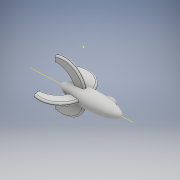
# Autodesk Inventor part: Rakete_Janneke
Saved by Autodesk Inventor 2017.3 (Build 213257000, 257)
## iProperties
Created: 2020-05-12
Part Number: Rakete_Janneke
Material: Generic
Document SubType Name: Modeling
Designer: Ole Simmering
Density: 1 g/cm^3
Appearance: Default
Author: Ole Simmering
Autodesk Inventor part; units mm, degrees
ref_plane "YZ Plane" through (0, 0, 0) normal (1, 0, 0) x (0, 1, 0)
ref_plane "XZ Plane" through (0, 0, 0) normal (0, 1, 0) x (-1, 0, 0)
ref_plane "XY Plane" through (0, 0, 0) normal (0, 0, 1) x (1, 0, 0)
sketch "Sketch1" plane through (0, 0, 0) normal (0, 0, 1) x (1, 0, 0)
  line L0 (23.379463, -14.591224) -> (429.779457, -14.591224) construction
  line L1 (429.779457, -14.591224) -> (429.779457, -319.391219) construction
  line L2 (429.779457, -319.391219) -> (23.379463, -319.391219) construction
  line L3 (23.379463, -319.391219) -> (23.379463, -14.591224) construction
  ellipse E0 centre (221, -186) end of major axis (94.610324, -191.310491) minor radius 34.213334 (347.389676, -180.689509) -> (94.610324, -191.310491) ccw
  line L4 (23.379463, -194.303384) -> (429.779457, -177.227754)
  ellipse E1 centre (221, -186) end of major axis (94.610324, -191.310491) minor radius 34.213334 (94.610324, -191.310491) -> (347.389676, -180.689509) ccw
  point P0 (0, 0)
  constraints: 4 point on line, 2 end point, 11 other
revolve "Revolution1" add sketch "Sketch1" angle 360 about axis through (23.379463, -194.303384, 0) along (0.9991185, 0.0419798, 0) contours L4 E0
sketch "Sketch3" plane through (0, 0, 0) normal (0, 0, 1) x (1, 0, 0)
  ellipse E0 centre (221, -186) end of major axis (94.610324, -191.310491) minor radius 34.213334 (347.389676, -180.689509) -> (94.610324, -191.310491) ccw construction
  arc A0 (147, -161.121791) -> (70, -117) centre (72.883013, -201.218571) ccw
  arc A1 (195, -153.503332) -> (70, -87) centre (103.165951, -175.388093) ccw
  line L0 (70, -87) -> (70, -117)
  line L1 (147, -161.121791) -> (176, -178)
  line L2 (176, -178) -> (195, -153.503332)
  point P0 (0, 0)
  constraints: 6 end point, 4 point on circle, 2 centre point, 1 vertical, 3 other
extrude "Extrusion1" add sketch "Sketch3" along normal mid plane 15
fillet "Fillet1" radius 7 4 edges at (147.5074, -92.0438, 7.5) (147.5074, -92.0438, -7.5) (114.7788, -128.1034, 7.5) (114.7788, -128.1034, -7.5)
sketch "Sketch4" plane through (0, 0, 0) normal (0, 0, 1) x (1, 0, 0)
  ellipse E0 centre (221, -186) end of major axis (94.610324, -191.310491) minor radius 34.213334 (347.389676, -180.689509) -> (195, -153.503332) ccw construction
  line L0 (347.389676, -180.689509) -> (94.610324, -191.310491) construction
  point P0 (0, 0)
  constraints: 2 end point, 3 other
pattern_circular "Circular Pattern1" count 4 over 360 about axis through (347.389676, -180.689509, 0) along (-0.9991185, -0.0419798, 0) of "Extrusion1", "Fillet1"
sketch "Sketch5" plane through (0, 0, 0) normal (0, 0, 1) x (1, 0, 0)
  ellipse E0 centre (221, -186) end of major axis (94.610324, -191.310491) minor radius 34.213334 (347.389676, -180.689509) -> (195, -153.503332) ccw
  ellipse E1 centre (266.909611, -152.309547) end of major axis (240.109303, -153.43561) minor radius 16.399914 (240.228627, -151.4085) -> (240.125165, -152.309547) ccw
  line L0 (240.125165, -152.309547) -> (293.694057, -152.309547)
  ellipse E2 centre (266.909611, -152.309547) end of major axis (240.109303, -153.43561) minor radius 16.399914 (293.694057, -152.309547) -> (240.228627, -151.4085) ccw
  ellipse E3 centre (266.909611, -152.309547) end of major axis (240.109303, -153.43561) minor radius 16.399914 (240.125165, -152.309547) -> (293.694057, -152.309547) ccw
  point P0 (0, 0)
  constraints: 2 end point, 1 horizontal, 1 midpoint, 15 other
revolve "Revolution2" add sketch "Sketch5" angle 360 about axis through (240.125165, -152.309547, 0) along (1, 0, 0) contours E0 E2 L0
body "Solid1"
